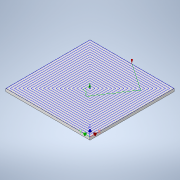
# Autodesk Inventor part: CNC_bed_face
Saved by Autodesk Inventor 2020 (Build 240168000, 168)
## iProperties
Created: 2021-10-16
Part Number: CNC_bed_face
Material: 一般
Document SubType Name: Modeling
Designer: naoki
Density: 1 g/cm^3
Appearance: 既定
Author: naoki
Autodesk Inventor part; units mm, degrees
ref_plane "YZ Plane" through (0, 0, 0) normal (1, 0, 0) x (0, 1, 0)
ref_plane "XZ Plane" through (0, 0, 0) normal (0, 1, 0) x (-1, 0, 0)
ref_plane "XY Plane" through (0, 0, 0) normal (0, 0, 1) x (1, 0, 0)
sketch "スケッチ2" plane through (0, 0, 0) normal (0, 0, 1) x (1, 0, 0)
  line L0 (-150, -150) -> (150, -150)
  line L1 (150, -150) -> (150, 150)
  line L2 (150, 150) -> (-150, 150)
  line L3 (-150, 150) -> (-150, -150)
  line L4 (-150, -150) -> (150, 150) construction
  line L5 (150, -150) -> (-150, 150) construction
  point P0 (0, 0)
  dimension "d4" = 300
  dimension "d5" = 300
  constraints: 12 end point, 2 midpoint, 2 parallel, 1 horizontal, 1 perpendicular
  measures "d4" distance of L2.end L1.end
  measures "d5" distance of L1.end L0.end
extrude "押し出し1" add sketch "スケッチ2" along normal blind 10
